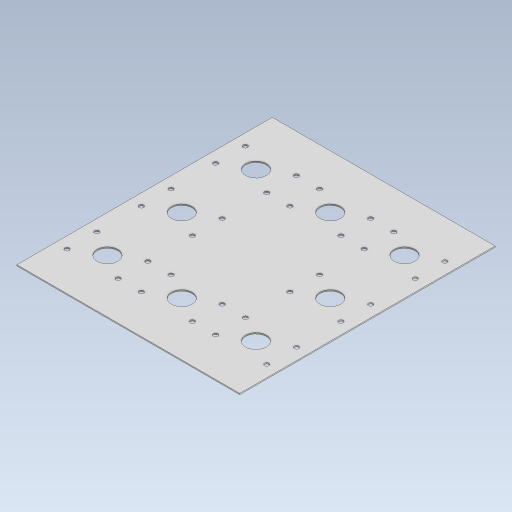
# Autodesk Inventor part: BasePlate
Saved by Autodesk Inventor 2023 (Build 270158000, 158)
## iProperties
Created: 2022-12-01
Part Number: BasePlate
Material: Generic
Document SubType Name: Modeling
Designer: Dave
Density: 1 g/cm^3
Appearance: Default
Author: Dave
Autodesk Inventor part; units mm, degrees
ref_plane "YZ Plane" through (0, 0, 0) normal (1, 0, 0) x (0, 1, 0)
ref_plane "XZ Plane" through (0, 0, 0) normal (0, 1, 0) x (-1, 0, 0)
ref_plane "XY Plane" through (0, 0, 0) normal (0, 0, 1) x (1, 0, 0)
sketch "Sketch1" plane through (0, 0, 0) normal (0, 1, 0) x (-1, 0, 0)
  line L0 (0, 0) -> (304.8, 0)
  line L1 (304.8, 0) -> (304.8, -349.25)
  line L2 (304.8, -349.25) -> (0, -349.25)
  line L3 (0, -349.25) -> (0, 0)
  dimension "d0" = 304.8
  dimension "d1" = 349.25
  constraints: 8 end point, 2 parallel, 1 horizontal, 1 perpendicular
  measures "d0" distance of L1.end L2.end
  measures "d1" distance of L0.end L1.end
extrude "Extrusion1" add sketch "Sketch1" along normal blind 1.5875
sketch "Sketch2" plane through (0, 1.5875, 0) normal (0, 1, 0) x (1, 0, 0)
  circle A0 centre (-254, 73.025) radius 14.2875
  line L0 (0, 349.25) -> (-304.8, 349.25) projected
  line L1 (-304.8, 349.25) -> (-304.8, 0) projected
  line L2 (-304.8, 0) -> (0, 0) projected
  line L3 (0, 0) -> (0, 349.25) projected
  circle A1 centre (-288.925, 52.705) radius 3.175
  circle A2 centre (-288.925, 93.345) radius 3.175
  circle A3 centre (-219.075, 93.345) radius 3.175
  circle A4 centre (-219.075, 52.705) radius 3.175
  line L4 (-254, 119.7319) -> (-254, 73.025) construction
  line L5 (-254, 73.025) -> (-226.8959, 73.025) construction
  line L6 (-304, 48.025) -> (-204, 48.025) construction
  line L7 (-204, 48.025) -> (-204, 98.025) construction
  line L8 (-204, 98.025) -> (-304, 98.025) construction
  line L9 (-304, 98.025) -> (-304, 48.025) construction
  line L10 (-304.8, 41.275) -> (0, 41.275)
  line L11 (0, 41.275) -> (0, 307.975)
  line L12 (0, 307.975) -> (-304.8, 307.975)
  line L13 (-304.8, 307.975) -> (-304.8, 41.275)
  line L14 (-202.4, 98.025) -> (-202.4, 48.025) construction
  circle A5 centre (-187.325, 93.345) radius 3.175
  circle A6 centre (-187.325, 52.705) radius 3.175
  circle A7 centre (-152.4, 73.025) radius 14.2875
  line L15 (-152.4, 73.025) -> (-125.2959, 73.025) construction
  line L16 (-152.4, 119.7319) -> (-152.4, 73.025) construction
  circle A8 centre (-117.475, 52.705) radius 3.175
  line L17 (-102.4, 48.025) -> (-102.4, 98.025) construction
  line L18 (-102.4, 98.025) -> (-202.4, 98.025) construction
  line L19 (-202.4, 48.025) -> (-102.4, 48.025) construction
  circle A9 centre (-117.475, 93.345) radius 3.175
  line L20 (-100.8, 98.025) -> (-100.8, 48.025) construction
  circle A10 centre (-85.725, 93.345) radius 3.175
  circle A11 centre (-85.725, 52.705) radius 3.175
  circle A12 centre (-50.8, 73.025) radius 14.2875
  line L21 (-50.8, 73.025) -> (-23.6959, 73.025) construction
  line L22 (-50.8, 119.7319) -> (-50.8, 73.025) construction
  circle A13 centre (-15.875, 52.705) radius 3.175
  line L23 (-0.8, 48.025) -> (-0.8, 98.025) construction
  line L24 (-0.8, 98.025) -> (-100.8, 98.025) construction
  line L25 (-100.8, 48.025) -> (-0.8, 48.025) construction
  circle A14 centre (-15.875, 93.345) radius 3.175
  line L26 (-304, 199.625) -> (-304, 149.625) construction
  circle A15 centre (-288.925, 194.945) radius 3.175
  circle A16 centre (-288.925, 154.305) radius 3.175
  circle A17 centre (-254, 174.625) radius 14.2875
  line L27 (-254, 174.625) -> (-226.8959, 174.625) construction
  line L28 (-254, 221.3319) -> (-254, 174.625) construction
  circle A18 centre (-219.075, 154.305) radius 3.175
  line L29 (-204, 149.625) -> (-204, 199.625) construction
  line L30 (-204, 199.625) -> (-304, 199.625) construction
  line L31 (-304, 149.625) -> (-204, 149.625) construction
  circle A19 centre (-219.075, 194.945) radius 3.175
  line L32 (-202.4, 199.625) -> (-202.4, 149.625) construction
  circle A20 centre (-187.325, 194.945) radius 3.175
  circle A21 centre (-187.325, 154.305) radius 3.175
  circle A22 centre (-152.4, 174.625) radius 14.2875
  line L33 (-152.4, 174.625) -> (-125.2959, 174.625) construction
  line L34 (-152.4, 221.3319) -> (-152.4, 174.625) construction
  circle A23 centre (-117.475, 154.305) radius 3.175
  line L35 (-102.4, 149.625) -> (-102.4, 199.625) construction
  line L36 (-102.4, 199.625) -> (-202.4, 199.625) construction
  line L37 (-202.4, 149.625) -> (-102.4, 149.625) construction
  circle A24 centre (-117.475, 194.945) radius 3.175
  line L38 (-100.8, 199.625) -> (-100.8, 149.625) construction
  circle A25 centre (-85.725, 194.945) radius 3.175
  circle A26 centre (-85.725, 154.305) radius 3.175
  circle A27 centre (-50.8, 174.625) radius 14.2875
  line L39 (-50.8, 174.625) -> (-23.6959, 174.625) construction
  line L40 (-50.8, 221.3319) -> (-50.8, 174.625) construction
  circle A28 centre (-15.875, 154.305) radius 3.175
  line L41 (-0.8, 149.625) -> (-0.8, 199.625) construction
  line L42 (-0.8, 199.625) -> (-100.8, 199.625) construction
  line L43 (-100.8, 149.625) -> (-0.8, 149.625) construction
  circle A29 centre (-15.875, 194.945) radius 3.175
  line L44 (-304, 301.225) -> (-304, 251.225) construction
  circle A30 centre (-288.925, 296.545) radius 3.175
  circle A31 centre (-288.925, 255.905) radius 3.175
  circle A32 centre (-254, 276.225) radius 14.2875
  line L45 (-254, 276.225) -> (-226.8959, 276.225) construction
  line L46 (-254, 322.9319) -> (-254, 276.225) construction
  circle A33 centre (-219.075, 255.905) radius 3.175
  line L47 (-204, 251.225) -> (-204, 301.225) construction
  line L48 (-204, 301.225) -> (-304, 301.225) construction
  line L49 (-304, 251.225) -> (-204, 251.225) construction
  circle A34 centre (-219.075, 296.545) radius 3.175
  line L50 (-202.4, 301.225) -> (-202.4, 251.225) construction
  circle A35 centre (-187.325, 296.545) radius 3.175
  circle A36 centre (-187.325, 255.905) radius 3.175
  circle A37 centre (-152.4, 276.225) radius 14.2875
  line L51 (-152.4, 276.225) -> (-125.2959, 276.225) construction
  line L52 (-152.4, 322.9319) -> (-152.4, 276.225) construction
  circle A38 centre (-117.475, 255.905) radius 3.175
  line L53 (-102.4, 251.225) -> (-102.4, 301.225) construction
  line L54 (-102.4, 301.225) -> (-202.4, 301.225) construction
  line L55 (-202.4, 251.225) -> (-102.4, 251.225) construction
  circle A39 centre (-117.475, 296.545) radius 3.175
  line L56 (-100.8, 301.225) -> (-100.8, 251.225) construction
  circle A40 centre (-85.725, 296.545) radius 3.175
  circle A41 centre (-85.725, 255.905) radius 3.175
  circle A42 centre (-50.8, 276.225) radius 14.2875
  line L57 (-50.8, 276.225) -> (-23.6959, 276.225) construction
  line L58 (-50.8, 322.9319) -> (-50.8, 276.225) construction
  circle A43 centre (-15.875, 255.905) radius 3.175
  line L59 (-0.8, 251.225) -> (-0.8, 301.225) construction
  line L60 (-0.8, 301.225) -> (-100.8, 301.225) construction
  line L61 (-100.8, 251.225) -> (-0.8, 251.225) construction
  circle A44 centre (-15.875, 296.545) radius 3.175
  point P0 (-304, 73.025)
  point P1 (-254, 98.025)
  point P2 (-304.8, 174.625)
  point P3 (-202.4, 73.025)
  point P4 (-152.4, 98.025)
  point P5 (-100.8, 73.025)
  point P6 (-50.8, 98.025)
  point P7 (-304, 174.625)
  point P8 (-254, 199.625)
  point P9 (-202.4, 174.625)
  point P10 (-152.4, 199.625)
  point P11 (-100.8, 174.625)
  point P12 (-50.8, 199.625)
  point P13 (-304, 276.225)
  point P14 (-254, 301.225)
  point P15 (-202.4, 276.225)
  point P16 (-152.4, 301.225)
  point P17 (-100.8, 276.225)
  point P18 (-50.8, 301.225)
  dimension "d4" = 28.575
  dimension "d5" = 6.35
  dimension "d6" = 20.32
  dimension "d7" = 34.925
  dimension "d8" = 50.8
  dimension "d9" = 100
  dimension "d10" = 50
  dimension "d11" = 266.7
  dimension "d12" = 31.75
  dimension "d15" = 101.6
  dimension "d18" = 101.6
  constraints: 116 end point, 45 centre point, 4 horizontal, 4 midpoint, 4 parallel, 3 equal radius, 2 perpendicular, 2 point on line, 1 horizontal alignment, 1 vertical, 1 vertical alignment, 196 other
  measures "d4" diameter of A0
  measures "d5" diameter of A2
  measures "d6" vertical distance of A1.centre L4.end
  measures "d7" horizontal distance of A4.centre L4.end
  measures "d8" distance from line of L1 L4.end
  measures "d9" distance of L8.end L7.end
  measures "d10" distance of L7.end L6.end
  measures "d11" distance of L12.end L10.start
  measures "d12" distance from line of L10 L4.end
  measures "d15" distance of A2.centre A5.centre
  measures "d18" distance of A2.centre A15.centre
extrude "Extrusion2" cut sketch "Sketch2" against normal through all contours A0 | A1 | A2 | A3 | A4 | A5 | A6 | A7 | A8 | A9 | A10 | A11 | A12 | A13 | A14 | A15 | A16 | A17 | A18 | A19 | A25 | A26 | A27 | A28 | A29 | A30 | A31 | A32 | A33 | A34 | A35 | A36 | A37 | A38 | A39 | A40 | A41 | A42 | A43 | A44
body "Solid1"
